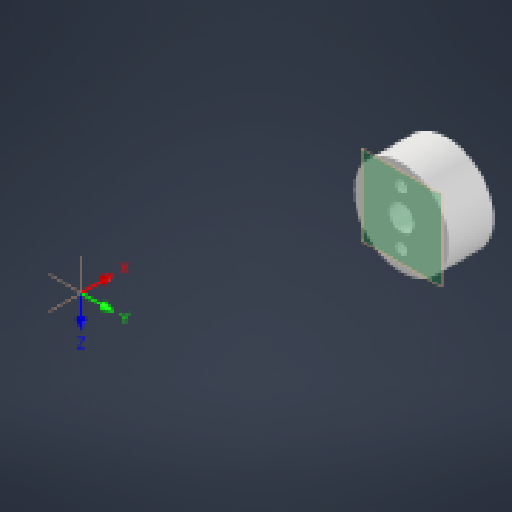
# Autodesk Inventor part: Knuckle
Saved by Autodesk Inventor 2025 (Build 290162000, 162)
## iProperties
Created: 2024-10-13
Part Number: Knuckle
Material: Типовые
Document SubType Name: Modeling
Designer: khrip
Density: 1 g/cm^3
Appearance: По умолчанию
Author: khrip
Autodesk Inventor part; units mm, degrees
ref_plane "YZ Plane" through (0, 0, 0) normal (1, 0, 0) x (0, 1, 0)
ref_plane "XZ Plane" through (0, 0, 0) normal (0, 1, 0) x (-1, 0, 0)
ref_plane "XY Plane" through (0, 0, 0) normal (0, 0, 1) x (1, 0, 0)
ref_plane "РабПлоскость1" through (0, 7.4, 15) normal (0, 0, -1) x (-1, 0, 0)
sketch "Эскиз1" plane through (0, 7.4, 15) normal (0, 0, -1) x (-1, 0, 0)
  circle A0 centre (0, 0) radius 12.5
  circle A1 centre (0, 0) radius 12.5 projected
  circle A2 centre (0, -8.5) radius 1.2295 projected
  circle A3 centre (0, 8.5) radius 1.2295 projected
  circle A4 centre (0, 0) radius 3.5 projected
  circle A5 centre (0, 0) radius 4
  circle A6 centre (0, 0) radius 15
  circle A7 centre (0, 0) radius 12.7
  point P0 (0, -7.4)
  dimension "d6" = 0
  dimension "d7" = 0
  dimension "d8" = 0
  dimension "d9" = 8
  dimension "d10" = 30
  dimension "d11" = 0.2
  constraints: 4 centre point, 3 coincident
  measures "d6" radial gap between concentric circles of A1 A0
  measures "d7" distance of A1.centre A0.centre
  measures "d8" distance of A1.centre A0.centre
  measures "d9" diameter of A5
  measures "d10" diameter of A6
  measures "d11" radial gap between concentric circles of A7 A0
extrude "Выдавливание1" add sketch "Эскиз1" along normal blind 2.5 contours A0 | A6 | A7
sketch "Эскиз2" plane through (0, 7.4, 12.5) normal (0, 0, -1) x (-1, 0, 0)
  circle A0 centre (0, 0) radius 15 projected
  circle A1 centre (0, -8.5) radius 1.2295 projected
  circle A2 centre (0, 8.5) radius 1.2295 projected
  circle A3 centre (0, 0) radius 4 projected
  point P0 (0, -7.4)
  constraints: 1 coincident
hole "Отверстие1" at (0, -1.1, 12.5) at (0, 15.9, 12.5) direction (0, 0, 1) diameter 3.4 end through all countersink diameter 6.6 countersink angle 90 clearance for "с потайной головкой ГОСТ 12876-67" size "M3" standard "ГОСТ"
sketch "Эскиз3" plane through (0, 7.4, 12.5) normal (0, 0, -1) x (-1, 0, 0)
  circle A0 centre (0, 0) radius 5 projected
  circle A1 centre (0, 0) radius 10.5 projected
  circle A2 centre (0, 0) radius 15 projected
  circle A3 centre (0, -8.5) radius 3.3 projected
  circle A4 centre (0, 8.5) radius 3.3 projected
  circle A5 centre (0, -8.5) radius 3.3 projected
  circle A6 centre (0, 0) radius 15 projected
  circle A7 centre (0, 0) radius 4 projected
  circle A8 centre (0, 0) radius 5.5
  point P0 (0, -7.4)
  point P1 (-1.1003, -5.3888)
  point P2 (-1.1003, 5.3888)
  point P3 (1.1003, 5.3888)
  point P4 (1.1003, -5.3888)
  dimension "d21" = 11
  constraints: 1 centre point, 1 coincident
  measures "d21" diameter of A8
extrude "Выдавливание2" add sketch "Эскиз3" along normal blind 6 contours A1 A3 A8 A4 | A4 A8 A3 A1 | A2
sketch "Эскиз4" plane through (0, 7.4, 6.5) normal (0, 0, -1) x (-1, 0, 0)
  circle A0 centre (0, 0) radius 15 projected
  arc A1 (-1.1003, 5.3888) -> (-1.1003, -5.3888) centre (0, 0) ccw projected
  arc A2 (1.1003, 5.3888) -> (-1.1003, 5.3888) centre (0, 8.5) ccw projected
  arc A3 (1.1003, -5.3888) -> (1.1003, 5.3888) centre (0, 0) ccw projected
  arc A4 (-1.1003, -5.3888) -> (1.1003, -5.3888) centre (0, -8.5) ccw projected
  arc A5 (-7.599, -4.8836) -> (-3.7524, -8.2167) centre (0, 0) ccw projected
  circle A6 centre (0, 0) radius 10.5 projected
  circle A7 centre (0, 0) radius 9.033
  point P0 (0, -7.4)
  point P1 (-3.2987, -8.4091)
  point P2 (-3.7524, -8.2167)
  point P3 (-7.599, -4.8836)
  point P4 (-3.2987, 8.4091)
  point P5 (3.2987, 8.4091)
  point P6 (3.2987, -8.4091)
  constraints: 1 centre point, 1 coincident, 1 concentric
ref_plane "РабПлоскость2" through (-10.2, -2.8, 5.75) normal (0, 0, 1) x (1, 0, 0)
extrude "Выдавливание3" add sketch "Эскиз4" along normal up to surface (0.75 mm away) contours A0 | A7 A5 A4 A6 A2 | A2 A6 A4 A7
sketch "Эскиз5" plane through (0, 7.4, 5.75) normal (0, 0, -1) x (-1, 0, 0)
  arc A0 (-3.2987, -8.4091) -> (3.2987, -8.4091) centre (0, -8.5) ccw projected
  arc A1 (-3.2987, 8.4091) -> (-3.2987, -8.4091) centre (0, 0) ccw projected
  arc A2 (3.2987, 8.4091) -> (-3.2987, 8.4091) centre (0, 8.5) ccw projected
  arc A3 (3.2987, -8.4091) -> (3.2987, 8.4091) centre (0, 0) ccw projected
  circle A4 centre (0, 0) radius 15 projected
  circle A5 centre (0, 0) radius 10.5 projected
  point P0 (0, -7.4)
  point P1 (2.8891, 10.0947)
  point P2 (2.8891, -10.0947)
  point P3 (-2.8891, -10.0947)
  point P4 (-2.8891, 10.0947)
ref_plane "РабПлоскость3" through (-10.2, -2.8, 0.75) normal (0, 0, -1) x (0, 1, 0)
extrude "Выдавливание4" add sketch "Эскиз5" along normal up to surface (5 mm away)
